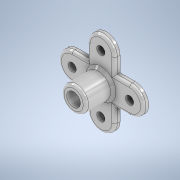
# Autodesk Inventor part: dudukan gps
Saved by Autodesk Inventor 2020 (Build 240168000, 168)
## iProperties
Created: 2020-01-30
Part Number: dudukan gps
Material: Generic
Document SubType Name: Modeling
Designer: Ferdi
Density: 1 g/cm^3
Appearance: Aluminum - Polished
Author: Ferdi
Autodesk Inventor part; units mm, degrees
ref_plane "YZ Plane" through (0, 0, 0) normal (1, 0, 0) x (0, 1, 0)
ref_plane "XZ Plane" through (0, 0, 0) normal (0, 1, 0) x (-1, 0, 0)
ref_plane "XY Plane" through (0, 0, 0) normal (0, 0, 1) x (1, 0, 0)
sketch "Sketch1" plane through (0, 0, 0) normal (0, 0, 1) x (1, 0, 0)
  circle A0 centre (0, 0) radius 2.5
  line L0 (0, 0) -> (-10.5, 0)
  circle A1 centre (-10.5, 0) radius 1.5
  arc A2 (-10.5, 5) -> (-10.5, -5) centre (-10.5, 0) ccw
  line L1 (-10.5, 5) -> (0, 5)
  line L2 (0, 5) -> (0, -5)
  line L3 (0, -5) -> (-10.5, -5)
  line L4 (0, 0) -> (0, -10.5)
  circle A3 centre (0, -10.5) radius 1.5
  arc A4 (-5, -10.5) -> (5, -10.5) centre (0, -10.5) ccw
  line L5 (-5, -10.5) -> (-5, 0)
  line L6 (5, 0) -> (5, -10.5)
  line L7 (0, 0) -> (10.5, 0)
  circle A5 centre (10.5, 0) radius 1.5
  arc A6 (10.5, -5) -> (10.5, 5) centre (10.5, 0) ccw
  line L8 (10.5, -5) -> (0, -5)
  line L9 (0, 5) -> (10.5, 5)
  line L10 (0, 0) -> (0, 10.5)
  circle A7 centre (0, 10.5) radius 1.5
  arc A8 (5, 10.5) -> (-5, 10.5) centre (0, 10.5) ccw
  line L11 (5, 10.5) -> (5, 0)
  line L12 (-5, 0) -> (-5, 10.5)
  circle A9 centre (0, 0) radius 4.5
  point P0 (-5, -5)
  point P1 (5, -5)
  point P2 (5, 5)
  point P3 (-5, 5)
  dimension "d0" = 10.5
  dimension "d1" = 3
  dimension "d2" = 5
  dimension "d3" = 10
  dimension "d6" = 360
  dimension "d8" = 9
  constraints: 26 end point, 10 centre point, 10 coincident, 8 point on circle, 2 horizontal, 1 parallel, 1 perpendicular, 53 other
  measures "d0" distance of L0.end L0.start
  measures "d1" diameter of A1
  measures "d2" diameter of A0
  measures "d3" diameter of A2
  measures "d8" diameter of A9
extrude "Extrusion1" add sketch "Sketch1" against normal blind 2 contours L7 A9 L2 A0 | A0 L2 A9 L7 | A0 L0 A9 L2 | L2 A9 L0 A0 | A9 L2 L9 L11 L7 | L7 L6 L8 L2 A9 | A9 L0 L12 L1 L2 | L2 L3 L5 L0 A9 | L11 L9 A6 L8 L6 | L1 L12 A8 L11 L9 | L8 L6 A4 L5 L3 | L5 L3 A2 L1 L12
extrude "Extrusion2" add sketch "Sketch1" along normal blind 10 contours L7 A9 L2 A0 | A0 L2 A9 L7 | A0 L0 A9 L2 | L2 A9 L0 A0
fillet "Fillet1" radius 1 12 edges at (-7.75, -5, 0) (-7.75, 5, 0) (-15.5, 0, 0) (5, -7.75, 0) (-5, -7.75, 0) (0, -15.5, 0) (15.5, 0, 0) (7.75, 5, 0) (7.75, -5, 0) (-5, 7.75, 0) (5, 7.75, 0) (0, 15.5, 0)
chamfer "Chamfer1" distance 1 angle 45 1 edges at (-4.5, 0, 0)
fillet "Fillet2" radius 1 1 edges at (-4.5, 0, 10)
body "Solid1"
